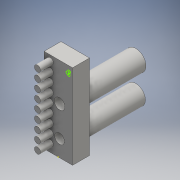
# Autodesk Inventor part: 0315_부품2
Saved by Autodesk Inventor 2016 (Build 200138000, 138)
## iProperties
Created: 2024-03-15
Part Number: 0315_부품2
Material: 일반
Document SubType Name: Modeling
Designer: pc
Density: 1 g/cm^3
Appearance: 기본값
Author: pc
Autodesk Inventor part; units mm, degrees
ref_plane "YZ Plane" through (0, 0, 0) normal (1, 0, 0) x (0, 1, 0)
ref_plane "XZ Plane" through (0, 0, 0) normal (0, 1, 0) x (-1, 0, 0)
ref_plane "XY Plane" through (0, 0, 0) normal (0, 0, 1) x (1, 0, 0)
sketch "스케치1" plane through (0, 0, 0) normal (0, 0, 1) x (1, 0, 0)
  line L0 (-16.8705, 10.0415) -> (16.8705, 10.0415)
  line L1 (16.8705, 10.0415) -> (16.8705, -10.0415)
  line L2 (16.8705, -10.0415) -> (-16.8705, -10.0415)
  line L3 (-16.8705, -10.0415) -> (-16.8705, 10.0415)
  line L4 (-16.8705, 10.0415) -> (16.8705, -10.0415) construction
  line L5 (16.8705, 10.0415) -> (-16.8705, -10.0415) construction
  point P0 (0, 0)
  constraints: 12 end point, 2 midpoint, 2 parallel, 1 horizontal, 1 perpendicular
extrude "돌출1" add sketch "스케치1" along normal blind 100
sketch "스케치2" plane through (-16.8705, 10.0415, 0) normal (0, 1, 0) x (1, 0, 0)
  circle A0 centre (18.3629, -19.7614) radius 11.3174
  circle A1 centre (18.3629, -55.0184) radius 11.9571
  point P0 (16.8705, 0)
  constraints: 2 centre point
extrude "돌출2" add sketch "스케치2" along normal blind 70.25
sketch "스케치3" plane through (1.4924, 80.2915, 19.7614) normal (0, 1, 0) x (1, 0, 0)
  circle A0 centre (0, 0) radius 5.7988
  circle A1 centre (0, -35.6989) radius 6.3
  point P0 (-1.4924, 19.7614)
  constraints: 2 centre point
extrude "돌출3" cut sketch "스케치3" against normal through all
sketch "스케치4" plane through (-16.8705, -10.0415, 0) normal (0, -1, 0) x (1, 0, 0)
  circle A0 centre (7.4206, 93.661) radius 3.6203
  point P0 (16.8705, 0)
  constraints: 1 centre point
extrude "돌출4" add sketch "스케치4" along normal blind 15.25
pattern_linear "직사각형 패턴1" count 9 spacing 10.5 along (0, 0, -1) of "돌출4"
sketch "스케치5" plane through (-16.8705, -10.0415, 0) normal (0, -1, 0) x (1, 0, 0)
  line L0 (27.8588, 94.265) -> (25.5194, 91.9257)
  line L1 (25.5194, 91.9257) -> (27.8178, 89.6273)
  arc A0 (27.8178, 89.6273) -> (27.8178, 91.969) centre (28.9886, 90.7982) ccw
  arc A1 (28.9886, 92.454) -> (27.8372, 93.9543) centre (29.4912, 94.0317) ccw
  arc A2 (29.6562, 92.7123) -> (28.9886, 92.454) centre (29.4017, 92.3783) ccw
  point P0 (16.8705, 0)
  constraints: 8 point on circle, 4 end point, 3 centre point, 1 perpendicular, 1 tangent
